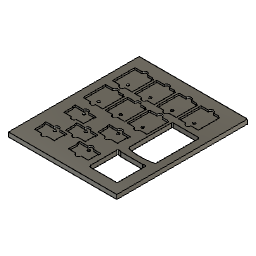
Pokemon_Shadow_Box_v12 (Autodesk Fusion 360 design; units mm, degrees)
Autodesk Fusion 360 part; units mm, degrees
note: some values were not read from the file. Set by a fixed rule: which sketch regions a step uses.
sketch "Sketch1" plane through (0, 0, 0) normal (0, 0, 1) x (1, 0, 0)
  line L0 (88.3497, -250.444) -> (31.4537, -250.444)
  line L1 (90.3975, -215.9) -> (90.3975, -223.012)
  line L2 (29.4058, -223.012) -> (29.4058, -215.9)
  line L3 (90.6515, -223.266) -> (88.6037, -223.266)
  line L4 (88.3497, -223.012) -> (88.3497, -250.444)
  line L5 (31.4537, -223.012) -> (29.4058, -223.012)
  circle A0 centre (59.9017, -215.9) radius 7.62
  line L6 (29.1518, -223.266) -> (29.1518, -215.646)
  line L7 (90.6515, -215.646) -> (90.6515, -223.266)
  line L8 (31.1997, -223.266) -> (29.1518, -223.266)
  line L9 (31.4537, -250.444) -> (31.4537, -223.012)
  line L10 (29.4058, -215.9) -> (90.3975, -215.9)
  line L11 (88.6037, -250.698) -> (31.1997, -250.698)
  line L12 (88.6037, -223.266) -> (88.6037, -250.698)
  circle A1 centre (59.9017, -250.444) radius 7.62
  line L13 (31.1997, -250.698) -> (31.1997, -223.266)
  line L14 (90.3975, -223.012) -> (88.3497, -223.012)
  line L15 (29.1518, -215.646) -> (90.6515, -215.646)
  circle A2 centre (59.9017, -220.2498) radius 3.9688
  line L16 (79.2575, -99.8855) -> (21.8535, -99.8855)
  line L17 (74.1775, -37.4015) -> (74.1775, -34.3535)
  line L18 (22.1075, -34.6075) -> (73.9235, -34.6075)
  line L19 (79.2575, -37.4015) -> (74.1775, -37.4015)
  line L20 (21.8535, -99.8855) -> (21.8535, -34.3535)
  line L21 (79.2575, -37.4015) -> (79.2575, -99.8855)
  line L22 (21.8535, -34.3535) -> (74.1775, -34.3535)
  line L23 (79.0035, -37.6555) -> (73.9235, -37.6555)
  line L24 (79.0035, -99.6315) -> (22.1075, -99.6315)
  line L25 (22.1075, -99.6315) -> (22.1075, -34.6075)
  line L26 (73.9235, -37.6555) -> (73.9235, -34.6075)
  circle A3 centre (50.5555, -83.1215) radius 3.9688
  line L27 (79.0035, -37.6555) -> (79.0035, -99.6315)
  line L28 (150.7458, -120.6182) -> (150.7458, -184.9755)
  line L29 (200.5298, -180.1495) -> (200.5298, -141.5415) construction
  line L30 (150.4918, -185.2295) -> (207.8958, -185.2295)
  line L31 (157.8578, -141.5415) -> (157.8578, -180.1495) construction
  arc A4 (207.8958, -120.3737) -> (150.4918, -120.3737) centre (179.1938, -870.0785) ccw
  line L32 (207.6418, -184.9755) -> (207.6418, -120.6182)
  line L33 (157.8578, -180.1495) -> (200.5298, -180.1495) construction
  line L34 (207.8958, -185.2295) -> (207.8958, -120.3737)
  line L35 (150.7458, -184.9755) -> (207.6418, -184.9755)
  line L36 (200.5298, -141.5415) -> (157.8578, -141.5415) construction
  circle A5 centre (179.1938, -168.4655) radius 3.9688
  line L37 (150.4918, -120.3737) -> (150.4918, -185.2295)
  arc A6 (207.6418, -120.6182) -> (150.7458, -120.6182) centre (179.1938, -870.0785) ccw
  line L38 (293.805, -246.2647) -> (293.805, -118.1735)
  line L39 (215.065, -118.1735) -> (215.065, -246.2647)
  arc A7 (215.065, -246.2647) -> (293.805, -246.2647) centre (254.435, -101.5235) ccw
  line L40 (276.279, -131.1275) -> (276.279, -184.9755) construction
  line L41 (293.805, -118.1735) -> (215.065, -118.1735)
  line L42 (276.279, -184.9755) -> (232.591, -184.9755) construction
  line L43 (232.591, -131.1275) -> (276.279, -131.1275) construction
  line L44 (232.591, -184.9755) -> (232.591, -131.1275) construction
  line L45 (213.1007, -267.589) -> (213.1007, -266.319)
  line L46 (286.5067, -350.647) -> (204.2107, -350.647)
  line L47 (204.2107, -350.647) -> (204.2107, -267.589)
  line L48 (204.2107, -267.589) -> (286.5067, -267.589)
  line L49 (286.5067, -266.319) -> (286.5067, -267.589)
  line L50 (286.5067, -267.589) -> (286.5067, -350.647)
  line L51 (204.2107, -267.589) -> (213.1007, -267.589)
  line L52 (245.3587, -267.589) -> (245.3587, -350.647) construction
  line L53 (204.2107, -266.319) -> (204.2107, -267.589)
  line L54 (213.1007, -266.319) -> (204.2107, -266.319)
  line L55 (277.6167, -267.589) -> (277.6167, -266.319)
  line L56 (277.6167, -266.319) -> (286.5067, -266.319)
  line L57 (0, 0) -> (315.9125, 0)
  line L58 (315.9125, 0) -> (315.9125, -381)
  line L59 (315.9125, -381) -> (0, -381)
  line L60 (0, -381) -> (0, 0)
  line L61 (301.2281, -14.2875) -> (14.6844, -14.2875)
  line L62 (14.6844, -14.2875) -> (14.6844, -366.7125)
  line L63 (14.6844, -366.7125) -> (301.2281, -366.7125)
  line L64 (301.2281, -366.7125) -> (301.2281, -14.2875)
  line L65 (143.3227, -37.6555) -> (138.2427, -37.6555)
  line L66 (86.4267, -99.6315) -> (86.4267, -34.6075)
  line L67 (143.3227, -37.6555) -> (143.3227, -99.6315)
  line L68 (138.2427, -37.6555) -> (138.2427, -34.6075)
  line L69 (86.1727, -34.3535) -> (138.4967, -34.3535)
  line L70 (143.5767, -99.8855) -> (86.1727, -99.8855)
  line L71 (138.4967, -37.4015) -> (138.4967, -34.3535)
  line L72 (143.3227, -99.6315) -> (86.4267, -99.6315)
  line L73 (86.4267, -34.6075) -> (138.2427, -34.6075)
  line L74 (86.1727, -99.8855) -> (86.1727, -34.3535)
  line L75 (143.5767, -37.4015) -> (138.4967, -37.4015)
  line L76 (143.5767, -37.4015) -> (143.5767, -99.8855)
  circle A8 centre (114.8747, -83.1215) radius 3.9688
  line L77 (207.6418, -37.6555) -> (202.5618, -37.6555)
  line L78 (150.7458, -99.6315) -> (150.7458, -34.6075)
  line L79 (207.6418, -37.6555) -> (207.6418, -99.6315)
  line L80 (202.5618, -37.6555) -> (202.5618, -34.6075)
  line L81 (150.4918, -34.3535) -> (202.8158, -34.3535)
  line L82 (207.8958, -99.8855) -> (150.4918, -99.8855)
  line L83 (202.8158, -37.4015) -> (202.8158, -34.3535)
  line L84 (207.6418, -99.6315) -> (150.7458, -99.6315)
  line L85 (150.7458, -34.6075) -> (202.5618, -34.6075)
  line L86 (150.4918, -99.8855) -> (150.4918, -34.3535)
  line L87 (207.8958, -37.4015) -> (202.8158, -37.4015)
  line L88 (207.8958, -37.4015) -> (207.8958, -99.8855)
  circle A9 centre (179.1938, -83.1215) radius 3.9688
  line L89 (79.0035, -122.9995) -> (73.9235, -122.9995)
  line L90 (22.1075, -184.9755) -> (22.1075, -119.9515)
  line L91 (79.0035, -122.9995) -> (79.0035, -184.9755)
  line L92 (73.9235, -122.9995) -> (73.9235, -119.9515)
  line L93 (21.8535, -119.6975) -> (74.1775, -119.6975)
  line L94 (79.2575, -185.2295) -> (21.8535, -185.2295)
  line L95 (74.1775, -122.7455) -> (74.1775, -119.6975)
  line L96 (79.0035, -184.9755) -> (22.1075, -184.9755)
  line L97 (22.1075, -119.9515) -> (73.9235, -119.9515)
  line L98 (21.8535, -185.2295) -> (21.8535, -119.6975)
  line L99 (79.2575, -122.7455) -> (74.1775, -122.7455)
  line L100 (79.2575, -122.7455) -> (79.2575, -185.2295)
  circle A10 centre (50.5555, -168.4655) radius 3.9688
  line L101 (136.1017, -265.938) -> (136.1017, -293.37)
  line L102 (137.8955, -258.572) -> (137.8955, -265.684)
  line L103 (76.9038, -265.684) -> (76.9038, -258.572)
  line L104 (78.9517, -265.684) -> (76.9038, -265.684)
  line L105 (135.8477, -293.116) -> (78.9517, -293.116)
  line L106 (137.8955, -265.684) -> (135.8477, -265.684)
  circle A11 centre (107.3997, -258.572) radius 7.62
  line L107 (76.6498, -258.318) -> (138.1495, -258.318)
  line L108 (136.1017, -293.37) -> (78.6977, -293.37)
  circle A12 centre (107.3997, -293.116) radius 7.62
  line L109 (76.6498, -265.938) -> (76.6498, -258.318)
  line L110 (76.9038, -258.572) -> (137.8955, -258.572)
  line L111 (78.9517, -293.116) -> (78.9517, -265.684)
  line L112 (135.8477, -265.684) -> (135.8477, -293.116)
  line L113 (78.6977, -265.938) -> (76.6498, -265.938)
  line L114 (78.6977, -293.37) -> (78.6977, -265.938)
  circle A13 centre (107.3997, -262.9217) radius 3.9688
  line L115 (138.1495, -258.318) -> (138.1495, -265.938)
  line L116 (138.1495, -265.938) -> (136.1017, -265.938)
  line L117 (271.961, -37.6555) -> (266.881, -37.6555)
  line L118 (215.065, -99.6315) -> (215.065, -34.6075)
  line L119 (271.961, -37.6555) -> (271.961, -99.6315)
  line L120 (266.881, -37.6555) -> (266.881, -34.6075)
  line L121 (214.811, -34.3535) -> (267.135, -34.3535)
  line L122 (272.215, -99.8855) -> (214.811, -99.8855)
  line L123 (267.135, -37.4015) -> (267.135, -34.3535)
  line L124 (271.961, -99.6315) -> (215.065, -99.6315)
  line L125 (215.065, -34.6075) -> (266.881, -34.6075)
  line L126 (214.811, -99.8855) -> (214.811, -34.3535)
  line L127 (272.215, -37.4015) -> (267.135, -37.4015)
  line L128 (272.215, -37.4015) -> (272.215, -99.8855)
  circle A14 centre (243.513, -83.1215) radius 3.9688
  line L129 (143.3227, -122.9995) -> (138.2427, -122.9995)
  line L130 (86.4267, -184.9755) -> (86.4267, -119.9515)
  line L131 (143.3227, -122.9995) -> (143.3227, -184.9755)
  line L132 (138.2427, -122.9995) -> (138.2427, -119.9515)
  line L133 (86.1727, -119.6975) -> (138.4967, -119.6975)
  line L134 (143.5767, -185.2295) -> (86.1727, -185.2295)
  line L135 (138.4967, -122.7455) -> (138.4967, -119.6975)
  line L136 (143.3227, -184.9755) -> (86.4267, -184.9755)
  line L137 (86.4267, -119.9515) -> (138.2427, -119.9515)
  line L138 (86.1727, -185.2295) -> (86.1727, -119.6975)
  line L139 (143.5767, -122.7455) -> (138.4967, -122.7455)
  line L140 (143.5767, -122.7455) -> (143.5767, -185.2295)
  circle A15 centre (114.8747, -168.4655) radius 3.9688
  line L141 (254.435, -251.5235) -> (254.435, -366.7125) construction
  circle A16 centre (158.9934, -215.9) radius 7.62
  line L142 (130.2914, -250.698) -> (130.2914, -223.266)
  line L143 (128.2435, -215.646) -> (189.7433, -215.646)
  circle A17 centre (158.9934, -220.2498) radius 3.9688
  line L144 (189.4893, -215.9) -> (189.4893, -223.012)
  line L145 (130.5454, -250.444) -> (130.5454, -223.012)
  line L146 (187.6954, -250.698) -> (130.2914, -250.698)
  line L147 (189.7433, -223.266) -> (187.6954, -223.266)
  line L148 (187.4414, -250.444) -> (130.5454, -250.444)
  line L149 (128.2435, -223.266) -> (128.2435, -215.646)
  line L150 (128.4975, -215.9) -> (189.4893, -215.9)
  line L151 (130.5454, -223.012) -> (128.4975, -223.012)
  line L152 (128.4975, -223.012) -> (128.4975, -215.9)
  line L153 (187.6954, -223.266) -> (187.6954, -250.698)
  line L154 (187.4414, -223.012) -> (187.4414, -250.444)
  line L155 (130.2914, -223.266) -> (128.2435, -223.266)
  line L156 (189.7433, -215.646) -> (189.7433, -223.266)
  circle A18 centre (158.9934, -250.444) radius 7.62
  line L157 (189.4893, -223.012) -> (187.4414, -223.012)
  circle A19 centre (59.9017, -301.244) radius 7.62
  line L158 (31.1997, -336.042) -> (31.1997, -308.61)
  line L159 (29.1518, -300.99) -> (90.6515, -300.99)
  circle A20 centre (59.9017, -305.5938) radius 3.9688
  line L160 (90.3975, -301.244) -> (90.3975, -308.356)
  line L161 (31.4537, -335.788) -> (31.4537, -308.356)
  line L162 (88.6037, -336.042) -> (31.1997, -336.042)
  line L163 (90.6515, -308.61) -> (88.6037, -308.61)
  line L164 (88.3497, -335.788) -> (31.4537, -335.788)
  line L165 (29.1518, -308.61) -> (29.1518, -300.99)
  line L166 (29.4058, -301.244) -> (90.3975, -301.244)
  line L167 (31.4537, -308.356) -> (29.4058, -308.356)
  line L168 (29.4058, -308.356) -> (29.4058, -301.244)
  line L169 (88.6037, -308.61) -> (88.6037, -336.042)
  line L170 (88.3497, -308.356) -> (88.3497, -335.788)
  line L171 (31.1997, -308.61) -> (29.1518, -308.61)
  line L172 (90.6515, -300.99) -> (90.6515, -308.61)
  circle A21 centre (59.9017, -335.788) radius 7.62
  line L173 (90.3975, -308.356) -> (88.3497, -308.356)
  circle A22 centre (158.9934, -301.244) radius 7.62
  line L174 (130.2914, -336.042) -> (130.2914, -308.61)
  line L175 (128.2435, -300.99) -> (189.7433, -300.99)
  circle A23 centre (158.9934, -305.5938) radius 3.9688
  line L176 (189.4893, -301.244) -> (189.4893, -308.356)
  line L177 (130.5454, -335.788) -> (130.5454, -308.356)
  line L178 (187.6954, -336.042) -> (130.2914, -336.042)
  line L179 (189.7433, -308.61) -> (187.6954, -308.61)
  line L180 (187.4414, -335.788) -> (130.5454, -335.788)
  line L181 (128.2435, -308.61) -> (128.2435, -300.99)
  line L182 (128.4975, -301.244) -> (189.4893, -301.244)
  line L183 (130.5454, -308.356) -> (128.4975, -308.356)
  line L184 (128.4975, -308.356) -> (128.4975, -301.244)
  line L185 (187.6954, -308.61) -> (187.6954, -336.042)
  line L186 (187.4414, -308.356) -> (187.4414, -335.788)
  line L187 (130.2914, -308.61) -> (128.2435, -308.61)
  line L188 (189.7433, -300.99) -> (189.7433, -308.61)
  circle A24 centre (158.9934, -335.788) radius 7.62
  line L189 (189.4893, -308.356) -> (187.4414, -308.356)
  line L190 (59.9017, -301.244) -> (59.9017, -250.444) construction
  line L191 (107.3997, -258.572) -> (107.3997, -293.116) construction
  line L192 (114.8747, -184.9755) -> (114.8747, -366.7125) construction
  circle A25 centre (50.5555, -34.6075) radius 7.62
  circle A26 centre (50.5555, -99.6315) radius 7.62
  circle A27 centre (114.8747, -34.6075) radius 7.62
  circle A28 centre (114.8747, -99.6315) radius 7.62
  circle A29 centre (179.1938, -34.6075) radius 7.62
  circle A30 centre (179.1938, -99.6315) radius 7.62
  circle A31 centre (243.513, -34.6075) radius 7.62
  circle A32 centre (243.513, -99.6315) radius 7.62
  circle A33 centre (50.5555, -119.9515) radius 7.62
  circle A34 centre (50.5555, -184.9755) radius 7.62
  circle A35 centre (114.8747, -119.9515) radius 7.62
  circle A36 centre (114.8747, -184.9755) radius 7.62
  circle A37 centre (179.1938, -119.9515) radius 7.62
  circle A38 centre (179.1938, -184.9755) radius 7.62
  arc A39 (214.811, -246.4587) -> (294.059, -246.4587) centre (254.435, -101.5235) ccw
  line L193 (294.059, -246.4587) -> (294.059, -117.9195)
  line L194 (294.059, -117.9195) -> (214.811, -117.9195)
  line L195 (214.811, -117.9195) -> (214.811, -246.4587)
  line L196 (203.9567, -267.335) -> (286.7607, -267.335)
  line L197 (286.7607, -267.335) -> (286.7607, -350.901)
  line L198 (286.7607, -350.901) -> (203.9567, -350.901)
  line L199 (203.9567, -350.901) -> (203.9567, -267.335)
  line L200 (277.3627, -267.589) -> (277.3627, -266.065)
  line L201 (277.3627, -266.065) -> (286.7607, -266.065)
  line L202 (286.7607, -266.065) -> (286.7607, -267.589)
  line L203 (203.9567, -267.843) -> (213.3547, -267.843)
  line L204 (213.3547, -267.843) -> (213.3547, -266.065)
  line L205 (213.3547, -266.065) -> (203.9567, -266.065)
  line L206 (203.9567, -266.065) -> (203.9567, -267.843)
  point P0 (59.9017, -215.9)
  point P1 (59.9017, -250.444)
  point P2 (59.9017, -216.281)
  point P3 (50.5555, -99.6315)
  point P4 (179.1938, -120.0785)
  point P5 (179.1938, -184.9755)
  point P6 (179.1938, -141.5415)
  point P7 (254.435, -251.5235)
  point P8 (254.435, -118.1735)
  point P9 (254.435, -131.1275)
  point P10 (157.9563, -366.7125)
  point P11 (157.9563, -381)
  point P12 (14.6844, -190.5)
  point P13 (0, -190.5)
  point P14 (114.8747, -99.6315)
  point P15 (179.1938, -99.6315)
  point P16 (50.5555, -184.9755)
  point P17 (107.3997, -258.572)
  point P18 (107.3997, -293.116)
  point P19 (107.3997, -258.953)
  point P20 (243.513, -99.6315)
  point P21 (114.8747, -184.9755)
  point P22 (254.435, -309.118)
  point P23 (245.3587, -309.118)
  point P24 (158.9934, -250.444)
  point P25 (158.9934, -215.9)
  point P26 (158.9934, -216.281)
  point P27 (59.9017, -335.788)
  point P28 (59.9017, -301.244)
  point P29 (59.9017, -301.625)
  point P30 (158.9934, -335.788)
  point P31 (158.9934, -301.244)
  point P32 (158.9934, -301.625)
  point P33 (107.3997, -275.844)
  point P34 (59.9017, -275.844)
  point P35 (114.8747, -275.844)
  point P36 (293.805, -34.6075)
  dimension "d2" = 56.896
  dimension "d3" = 34.544
  dimension "d4" = 7.112
  dimension "d5" = 60.9918
  dimension "d6" = 15.24
  dimension "d12" = 7.9375
  dimension "d14" = 0.254
  dimension "d15" = 65.024
  dimension "d16" = 51.816
  dimension "d17" = 61.976
  dimension "d18" = 56.896
  dimension "d19" = 7.9375
  dimension "d20" = 16.51
  dimension "d26" = 0.254
  dimension "d27" = 56.896
  dimension "d28" = 64.897
  dimension "d29" = 750
  dimension "d30" = 7.9375
  dimension "d31" = 16.51
  dimension "d36" = 43.434
  dimension "d37" = 4.826
  dimension "d38" = 7.112
  dimension "d39" = 78.74
  dimension "d40" = 150
  dimension "d41" = 133.35
  dimension "d46" = 66.802
  dimension "d47" = 12.954
  dimension "d48" = 17.526
  dimension "d49" = 82.296
  dimension "d50" = 83.058
  dimension "d51" = 84.328
  dimension "d52" = 8.89
  dimension "d53" = 315.9125
  dimension "d54" = 381
  dimension "d55" = 286.5438
  dimension "d56" = 352.425
  dimension "d59" = 64.3192
  dimension "d60" = 85.344
  dimension "d62" = 56.896
  dimension "d63" = 34.544
  dimension "d64" = 7.112
  dimension "d65" = 60.9918
  dimension "d66" = 15.24
  dimension "d67" = 7.9375
  dimension "d71" = 7.4231
  dimension "d72" = 7.4231
  dimension "d75" = 14.7214
  dimension "d76" = 14.7214
  dimension "d77" = 19.05
  dimension "d78" = 0.381
  dimension "d79" = 0.381
  dimension "d82" = 99.0918
  dimension "d83" = 85.344
  dimension "d86" = 20.32
  dimension "d87" = 15.24
  dimension "d88" = 15.24
  dimension "d89" = 15.24
  dimension "d90" = 15.24
  dimension "d91" = 0.254
  dimension "d94" = 0.254
  constraint vertical L4
  constraint perpendicular L0 L4
  constraint perpendicular L0 L9
  constraint perpendicular L5 L9
  constraint perpendicular L0 L2
  constraint perpendicular L2 L10
  constraint perpendicular L0 L1
  constraint perpendicular L4 L14
  constraint collinear L5 L14
  constraint midpoint P1 L0
  constraint midpoint P0 L10
  constraint vertical P0 P1
  constraint coincident P1 A1.centre
  constraint coincident P0 A0.centre
  constraint equal A0 A1
  constraint coincident A2 P2
  constraint vertical A2.centre P2
  constraint horizontal L18
  constraint vertical L27
  constraint horizontal L24
  constraint vertical L25
  constraint coincident L23.start L27
  constraint perpendicular L23 L27
  constraint coincident L26.end L18
  constraint perpendicular L18 L26
  constraint coincident L27.start L23
  constraint coincident L18.end L26
  constraint midpoint P3 L24
  constraint vertical A3.centre P3
  constraint vertical L28
  constraint perpendicular L28 L35
  constraint perpendicular L32 L35
  constraint horizontal L28.start L32.end
  constraint midpoint P4 A6
  constraint midpoint P5 L35
  constraint vertical P5 A5.centre
  constraint horizontal L36
  constraint vertical L31
  constraint horizontal L33
  constraint vertical L29
  constraint midpoint P6 L36
  constraint vertical P5 P6
  constraint vertical L38
  constraint perpendicular L38 L41
  constraint perpendicular L39 L41
  constraint horizontal L38.start L39.end
  constraint coincident P7 A7
  constraint midpoint P7 A7
  constraint horizontal L43
  constraint vertical L40
  constraint horizontal L42
  constraint vertical L44
  constraint midpoint P9 L43
  constraint midpoint P8 L41
  constraint vertical P8 P9
  constraint horizontal L48
  constraint vertical L50
  constraint horizontal L46
  constraint vertical L47
  constraint horizontal L51
  constraint vertical L45
  constraint horizontal L54
  constraint vertical L53
  constraint midpoint L52.start L48
  constraint midpoint L52.end L46
  constraint symmetric L47.end L48.end L52
  constraint symmetric L55.start L45.start L52
  constraint symmetric L55.end L45.end L52
  constraint symmetric L49.start L53.start L52
  constraint horizontal L57
  constraint vertical L58
  constraint horizontal L59
  constraint vertical L60
  constraint coincident L57.start L60.end
  constraint horizontal L61
  constraint vertical L62
  constraint horizontal L63
  constraint vertical L64
  constraint midpoint L63 P10
  constraint midpoint L59 P11
  constraint vertical P10 P11
  constraint midpoint L62 P12
  constraint midpoint L60 P13
  constraint horizontal P12 P13
  constraint vertical L112
  constraint perpendicular L105 L112
  constraint perpendicular L105 L111
  constraint perpendicular L104 L111
  constraint perpendicular L103 L105
  constraint perpendicular L103 L110
  constraint perpendicular L102 L105
  constraint perpendicular L106 L112
  constraint collinear L104 L106
  constraint midpoint P18 L105
  constraint midpoint P17 L110
  constraint vertical P17 P18
  constraint coincident P18 A12.centre
  constraint coincident P17 A11.centre
  constraint equal A11 A12
  constraint coincident P19 A13
  constraint vertical A13.centre P19
  constraint collinear L28 L78
  constraint collinear L35 L136
  constraint collinear L35 L42
  constraint coincident P7 L141.start
  constraint coincident L63 L141.end
  constraint perpendicular L63 L141
  constraint midpoint L141 P22
  constraint midpoint L52 P23
  constraint horizontal P22 P23
  constraint vertical P0 A2.centre
  constraint vertical P17 A13.centre
  constraint coincident P28 A19.centre
  constraint midpoint L191 P33
  constraint midpoint L190 P34
  constraint horizontal P33 P34
  constraint coincident P21 L192.start
  constraint coincident L63 L192.end
  constraint perpendicular L63 L192
  constraint midpoint L192 P35
  constraint horizontal P33 P35
  constraint coincident L18 A25.centre
  constraint vertical P3 A25.centre
  constraint coincident P3 A26.centre
  constraint coincident P5 A38.centre
  constraint vertical P4 A37.centre
  constraint horizontal A35.centre A37.centre
  constraint coincident L125 P36
  constraint coincident L38 P36
  measures "d2" distance of L0.end L0.start
  measures "d3" distance of L0 L10
  measures "d4" distance of L2.start L2.end
  measures "d5" distance of L1.start L2.end
  measures "d6" diameter of A0
  measures "d12" diameter of A2
  measures "d15" distance of L24.end L18.start
  measures "d16" distance of L25 L26
  measures "d17" distance of L23 L24
  measures "d18" distance of L25 L27
  measures "d19" diameter of A3
  measures "d20" distance of A3.centre P3
  measures "d27" distance of L28 L32
  measures "d28" distance of P4 L35
  measures "d29" radius of A6
  measures "d30" diameter of A5
  measures "d31" distance of A5.centre L35
  measures "d36" distance of L35 L36
  measures "d37" distance of L33 L35
  measures "d38" distance of L28 L31
  measures "d39" distance of L38 L39
  measures "d40" radius of A7
  measures "d41" distance of P7 L41
  measures "d46" distance of L41 L42
  measures "d47" distance of L41 L43
  measures "d48" distance of L39 L44
  measures "d49" distance of L47 L50
  measures "d50" distance of L46 L48
  measures "d51" distance of L46 L54
  measures "d52" distance of L45.end L53.start
  measures "d53" distance of L57.start L57.end
  measures "d54" distance of L57.start L59.end
  measures "d55" distance of L61.start L61.end
  measures "d56" distance of L61.end L62.end
  measures "d62" distance of L105.end L105.start
  measures "d63" distance of L105 L110
  measures "d64" distance of L103.end L103.start
  measures "d65" distance of L102.start L103.end
  measures "d66" diameter of A11
  measures "d67" diameter of A13
  measures "d71" distance of L25 L62
  measures "d72" distance of L32 L39
  measures "d75" distance of L50 L64
  measures "d76" distance of L2 L62
  measures "d77" distance of L4 P17
  measures "d78" distance of P17 P19
  measures "d79" distance of P0 P2
  measures "d86" distance of L18 L61
  measures "d87" diameter of A25
  measures "d88" diameter of A26
  measures "d89" diameter of A37
  measures "d90" diameter of A38
sketch "Sketch2" plane through (0, 0, 0) normal (0, 0, 1) x (1, 0, 0)
  line L0 (0, 0) -> (315.9125, 0)
  line L1 (315.9125, 0) -> (315.9125, -381)
  line L2 (315.9125, -381) -> (0, -381)
  line L3 (0, -381) -> (0, 0)
  line L4 (214.811, -117.9195) -> (214.811, -246.4587)
  arc A0 (214.811, -246.4587) -> (294.059, -246.4587) centre (254.435, -101.5235) ccw
  line L5 (294.059, -117.9195) -> (214.811, -117.9195)
  line L6 (294.059, -246.4587) -> (294.059, -117.9195)
  line L7 (286.7607, -267.335) -> (286.7607, -350.901)
  line L8 (286.7607, -350.901) -> (203.9567, -350.901)
  line L9 (203.9567, -350.901) -> (203.9567, -267.335)
  line L10 (203.9567, -266.065) -> (203.9567, -267.843)
  line L11 (213.3547, -266.065) -> (203.9567, -266.065)
  line L12 (213.3547, -267.843) -> (213.3547, -266.065)
  line L13 (203.9567, -267.335) -> (286.7607, -267.335)
  line L14 (277.3627, -267.589) -> (277.3627, -266.065)
  line L15 (277.3627, -266.065) -> (286.7607, -266.065)
  line L16 (286.7607, -266.065) -> (286.7607, -267.589)
extrude "Extrude1" add sketch "Sketch1" against normal blind 5.08 contours L57 L58 L59 L60 | L61 L62 L63 L64
extrude "Extrude2" add sketch "Sketch2" against normal blind 7.62 from surface at -5.08
extrude "Extrude3" cut sketch "Sketch1" against normal blind 3.175 from surface at -5.08 contours A0 A2 | A0 A2 | A3 | A5 | A8 | A9 | A10 | A11 A13 | A11 A13 | A14 | A15 | A16 A17 | A16 A17 | A19 A20 | A19 A20 | A22 A23 | A22 A23
fillet "Fillet1" radius 2.54 2 edges at (150.4918, -120.3737, -2.54) (207.8958, -120.3737, -2.54)
fillet "Fillet2" radius 2.54 4 edges at (294.059, -117.9195, -6.35) (214.811, -117.9195, -6.35) (203.9567, -266.065, -6.35) (286.7607, -266.065, -6.35)
fillet "Fillet3" radius 5.08 4 edges at (286.7607, -350.901, -6.35) (294.059, -246.4587, -6.35) (214.811, -246.4587, -6.35) (203.9567, -350.901, -6.35)
equation "d1 = -spacing"
equation "d2 = d62"
equation "d3 = d63"
equation "d4 = d64"
equation "d5 = d65"
equation "d6 = finger_dia"
equation "spacing = 0.01 in"
equation "d12 = magnet_dia"
equation "d14 = spacing"
equation "d19 = magnet_dia"
equation "magnet_dia = 0.3125 in"
equation "d26 = spacing"
equation "d30 = magnet_dia"
equation "d53 = 12 in + ( 7 / 16 ) * 1 in"
equation "d55 = 11 in + ( 4.5 / 16 ) * 1 in"
equation "d56 = 13 in + ( 14 / 16 ) * 1 in"
equation "d59 = top_game_spacing + d18"
equation "d60 = top_game_v_spacing + d15"
equation "d61 = -spacing"
equation "d66 = finger_dia"
equation "d67 = magnet_dia"
equation "finger_dia = 0.6 in"
equation "top_game_spacing = ( d55 - 2 * d18 - d27 - d39 ) / 5"
equation "d71 = top_game_spacing"
equation "d72 = top_game_spacing"
equation "gen3_h_space = 1.5 in"
equation "bottom_game_spacing = ( d55 - 2 * d65 - gen3_h_space - d49 ) / 3"
equation "d75 = bottom_game_spacing"
equation "d76 = bottom_game_spacing"
equation "d77 = gen3_h_space / 2"
equation "d79 = d78"
equation "d82 = gen3_h_space + d65"
equation "d83 = bottom_game_v_spacing + d63"
equation "bottom_game_v_spacing = 2 in"
equation "top_game_v_spacing = 0.8 in"
equation "d86 = top_game_v_spacing"
equation "d91 = spacing"
equation "d92 = -spacing"
equation "d93 = -spacing"
equation "d94 = spacing"
